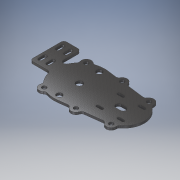
# Autodesk Inventor part: CAR REDUCTION PLATE I
Saved by Autodesk Inventor 2017 (Build 210142000, 142)
## iProperties
Part Number: CAR REDUCTION PLATE I
Material: Genérico
Document SubType Name: Modeling
Designer: Cristian
Density: 1 g/cm^3
Appearance: Valor por defecto
Author: Cristian
Autodesk Inventor part; units mm, degrees
ref_plane "YZ Plane" through (0, 0, 0) normal (1, 0, 0) x (0, 1, 0)
ref_plane "XZ Plane" through (0, 0, 0) normal (0, 1, 0) x (-1, 0, 0)
ref_plane "XY Plane" through (0, 0, 0) normal (0, 0, 1) x (1, 0, 0)
sketch "Boceto1" plane through (0, 0, 0) normal (0, 0, 1) x (1, 0, 0)
  circle A0 centre (0, 0) radius 57.15
  circle A1 centre (101.6, 0) radius 44.45
  circle A2 centre (-31.75, 47.519) radius 11.1125
  circle A3 centre (-31.75, -47.519) radius 11.1125
  circle A4 centre (114.3, 42.5971) radius 11.1125
  circle A5 centre (114.3, -42.5971) radius 11.1125
  line L0 (7.1437, 56.7018) -> (107.1562, 44.1014)
  circle A6 centre (44.45, 52.0016) radius 11.1125
  line L1 (7.1437, -56.7018) -> (107.1562, -44.1014)
  circle A7 centre (44.45, -52.0016) radius 11.1125
  dimension "d0" = 114.3
  dimension "d1" = 88.9
  dimension "d2" = 203.2
  dimension "d3" = 22.225
  dimension "d4" = 22.225
  dimension "d7" = 22.225
  dimension "d8" = 22.225
  dimension "d11" = 22.225
  dimension "d13" = 0
  dimension "d14" = 22.225
  dimension "d27" = 12.7
  dimension "d28" = 12.7
  dimension "d29" = 44.45
  dimension "d30" = 44.45
  dimension "d31" = 31.75
  dimension "d32" = 31.75
  constraints: 8 centre point, 8 point on circle, 4 end point, 4 tangent, 2 point on line, 1 coincident
  measures "d0" diameter of A0
  measures "d1" diameter of A1
  measures "d3" diameter of A2
  measures "d4" diameter of A3
  measures "d7" diameter of A4
  measures "d8" diameter of A5
  measures "d11" diameter of A6
  measures "d13" vertical distance of point (0, 0) A1.centre
  measures "d14" diameter of A7
  measures "d27" horizontal distance of A1.centre A4.centre
  measures "d28" horizontal distance of A1.centre A5.centre
  measures "d29" horizontal distance of point (0, 0) A6.centre
  measures "d30" horizontal distance of A7.centre point (0, 0)
  measures "d31" horizontal distance of point (0, 0) A2.centre
  measures "d32" horizontal distance of point (0, 0) A3.centre
extrude "Extrusión1" add sketch "Boceto1" along normal blind 5
sketch "Boceto2" plane through (0, 0, 5) normal (0, 0, 1) x (1, 0, 0)
  arc A0 (-21.9537, 52.7651) -> (-40.3458, 40.4764) centre (-31.75, 47.519) ccw projected
  circle A1 centre (-31.75, 47.519) radius 4.7625
  arc A2 (-40.3458, -40.4764) -> (-21.9537, -52.7651) centre (-31.75, -47.519) ccw projected
  circle A3 centre (-31.75, -47.519) radius 4.7625
  arc A4 (33.4247, -53.3907) -> (55.4753, -50.6125) centre (44.45, -52.0016) ccw projected
  circle A5 centre (44.45, -52.0016) radius 4.7625
  arc A6 (55.4753, 50.6125) -> (33.4247, 53.3907) centre (44.45, 52.0016) ccw projected
  circle A7 centre (44.45, 52.0016) radius 4.7625
  arc A8 (124.4689, 38.1158) -> (103.3657, 44.5789) centre (114.3, 42.5971) ccw projected
  circle A9 centre (114.3, 42.5971) radius 4.7625
  arc A10 (103.3657, -44.5789) -> (124.4689, -38.1158) centre (114.3, -42.5971) ccw projected
  circle A11 centre (114.3, -42.5971) radius 4.7625
  point P0 (0, 0)
  dimension "d18" = 9.525
  dimension "d19" = 9.525
  dimension "d20" = 9.525
  dimension "d21" = 9.525
  dimension "d22" = 9.525
  dimension "d23" = 9.525
  constraints: 6 centre point, 6 coincident
  measures "d18" diameter of A1
  measures "d19" diameter of A3
  measures "d20" diameter of A5
  measures "d21" diameter of A7
  measures "d22" diameter of A9
  measures "d23" diameter of A11
extrude "Extrusión2" cut sketch "Boceto2" against normal up to surface (5 mm away)
fillet "Empalme1" radius 6.35 12 edges at (-21.9537, -52.7651, 2.5) (-40.3458, -40.4764, 2.5) (33.4247, -53.3907, 2.5) (55.4753, -50.6125, 2.5) (124.4689, -38.1158, 2.5) (-40.3458, 40.4764, 2.5) (-21.9537, 52.7651, 2.5) (33.4247, 53.3907, 2.5) (55.4753, 50.6125, 2.5) (103.3657, 44.5789, 2.5) (124.4689, 38.1158, 2.5) (103.3657, -44.5789, 2.5)
sketch "Boceto3" plane through (0, 0, 0) normal (0, 0, -1) x (-1, 0, 0)
  circle A0 centre (0, 0) radius 7.1437
  circle A1 centre (0, -45) radius 6.35
  circle A2 centre (0, 45) radius 6.35
  line L0 (0, -45) -> (0, 0)
  line L1 (0, 0) -> (0, 45)
  dimension "d33" = 14.2875
  dimension "d34" = 12.7
  dimension "d35" = 12.7
  dimension "d36" = 45
  dimension "d37" = 45
  constraints: 4 end point, 3 centre point, 1 coincident, 1 collinear, 1 vertical
  measures "d33" diameter of A0
  measures "d34" diameter of A1
  measures "d35" diameter of A2
  measures "d36" distance of point (0, 0) L0.start
  measures "d37" distance of L1.end point (0, 0)
extrude "Extrusión3" cut sketch "Boceto3" against normal up to surface (5 mm away)
sketch "Boceto4" plane through (0, 0, 5) normal (0, 0, 1) x (1, 0, 0)
  circle A0 centre (93.4212, 0) radius 6.35
  line L0 (65.4212, -28) -> (121.4212, -28)
  line L1 (121.4212, -28) -> (121.4212, 28)
  line L2 (121.4212, 28) -> (65.4212, 28)
  line L3 (65.4212, 28) -> (65.4212, -28)
  line L4 (69.6712, -23.75) -> (117.1712, -23.75)
  line L5 (117.1712, -23.75) -> (117.1712, 23.75)
  line L6 (117.1712, 23.75) -> (69.6712, 23.75)
  line L7 (69.6712, 23.75) -> (69.6712, -23.75)
  circle A1 centre (74.8306, -23.75) radius 2.7781
  circle A2 centre (112.0118, -23.75) radius 2.7781
  circle A3 centre (122.3306, -23.75) radius 2.7781
  circle A4 centre (64.5118, -23.75) radius 2.7781
  line L8 (64.5118, -26.5281) -> (74.8306, -26.5281)
  line L9 (64.5118, -20.9719) -> (74.8306, -20.9719)
  line L10 (112.0118, -26.5281) -> (122.3306, -26.5281)
  line L11 (122.3306, -20.9719) -> (112.0118, -20.9719)
  circle A5 centre (74.8306, 23.75) radius 2.7781
  circle A6 centre (64.5118, 23.75) radius 2.7781
  line L12 (64.5118, 20.9719) -> (74.8306, 20.9719)
  line L13 (64.5118, 26.5281) -> (74.8306, 26.5281)
  circle A7 centre (112.0118, 23.75) radius 2.7781
  circle A8 centre (122.3306, 23.75) radius 2.7781
  line L14 (112.0118, 20.9719) -> (122.3306, 20.9719)
  line L15 (112.0118, 26.5281) -> (122.3306, 26.5281)
  circle A9 centre (98.5806, 0) radius 6.35
  circle A10 centre (88.2618, 0) radius 6.35
  line L16 (98.5806, 6.35) -> (88.2618, 6.35)
  line L17 (98.5806, -6.35) -> (88.2618, -6.35)
  point P0 (0, 0)
  dimension "d40" = 12.7
  dimension "d41" = 56
  dimension "d42" = 56
  dimension "d43" = 28
  dimension "d44" = 28
  dimension "d45" = 0
  dimension "d46" = 93.4212
  dimension "d47" = 47.5
  dimension "d48" = 47.5
  dimension "d49" = 23.75
  dimension "d50" = 23.75
  dimension "d57" = 5.5563
  dimension "d58" = 5.1594
  dimension "d59" = 5.5563
  dimension "d60" = 5.5563
  dimension "d61" = 5.1594
  dimension "d62" = 5.1594
  dimension "d63" = 5.5563
  dimension "d64" = 5.1594
  dimension "d65" = 0
  dimension "d66" = 5.5563
  dimension "d67" = 5.5563
  dimension "d68" = 5.1594
  dimension "d69" = 5.1594
  dimension "d70" = 0
  dimension "d71" = 5.5563
  dimension "d72" = 5.5563
  dimension "d73" = 5.1594
  dimension "d74" = 5.1594
  dimension "d75" = 0
  dimension "d78" = 12.7
  dimension "d79" = 12.7
  dimension "d80" = 5.1594
  dimension "d81" = 5.1594
  constraints: 36 end point, 20 point on circle, 20 tangent, 11 centre point, 5 point on line, 4 parallel, 2 horizontal, 2 perpendicular
  measures "d40" diameter of A0
  measures "d41" distance of L2.end L0.start
  measures "d42" distance of L1.end L2.end
  measures "d43" distance from line of L2 A0.centre
  measures "d44" distance from line of L3 A0.centre
  measures "d45" vertical distance of point (0, 0) A0.centre
  measures "d46" distance of point (0, 0) A0.centre
  measures "d47" distance of L6.end L4.start
  measures "d48" distance of L4.start L4.end
  measures "d49" distance from line of L4 A0.centre
  measures "d50" distance from line of L7 A0.centre
  measures "d57" diameter of A1
  measures "d58" distance of A1.centre L4.start
  measures "d59" diameter of A2
  measures "d60" diameter of A3
  measures "d61" distance of L4.end A2.centre
  measures "d62" distance of L4.end A3.centre
  measures "d63" diameter of A4
  measures "d64" distance of L4.start A4.centre
  measures "d65" distance from line of L4 A4.centre
  measures "d66" diameter of A5
  measures "d67" diameter of A6
  measures "d68" distance of L6.end A6.centre
  measures "d69" distance of L6.end A5.centre
  measures "d70" distance from line of L6 A6.centre
  measures "d71" diameter of A7
  measures "d72" diameter of A8
  measures "d73" distance of L5.end A7.centre
  measures "d74" distance of L5.end A8.centre
  measures "d75" distance from line of L6 A8.centre
  measures "d78" diameter of A9
  measures "d79" diameter of A10
  measures "d80" distance of A0.centre A9.centre
  measures "d81" distance of A0.centre A10.centre
extrude "Extrusión4" cut sketch "Boceto4" against normal up to next contours A0 A9 A10 | A0 A9 | A9 A10 A0 | A0 L16 A9 | A9 L17 A0 | A0 A10 A9 | A0 A10 L16 | A10 A9 | A9 A10 A0 | L17 A10 A0 | A0 A10 | L8 A4 L3 | L3 A4 L9 L7 L4 A1 L8 | L10 A2 L4 L5 L11 L1 A3 | L1 A3 L10 | A4 L3 | L3 A4 | A1 L4 | A3 L1 | L1 A3 | A2 L4 | A4 L9 L3 | L4 A1 | L4 L7 L9 A1 | L1 L11 A3 | A2 L11 L5 L4 | L4 A2 | L12 A6 L3 | L3 A6 L13 A5 L6 L7 L12 | L14 L5 L6 A7 L15 L1 A8 | L1 A8 L14 | A6 L3 | L3 A6 | L7 L6 A5 L12 | A8 L1 | L1 A8 | L14 A7 L6 L5 | A6 L13 L3 | A5 L6 | L1 L15 A8 | A7 L6 | A5 L6 | L6 A7
sketch "Boceto5" plane through (0, 0, 5) normal (0, 0, 1) x (1, 0, 0)
  line L0 (-101.6, -9.525) -> (-63.5, -9.525)
  line L1 (-63.5, -9.525) -> (-63.5, 66.675)
  line L2 (-63.5, 66.675) -> (-101.6, 66.675)
  line L3 (-101.6, 66.675) -> (-101.6, -9.525)
  arc A0 (127.9228, -35.8178) -> (127.9228, 35.8178) centre (101.6, 0) ccw projected
  line L4 (146.05, 0) -> (146.05, -41.4145)
  arc A1 (-17.8783, -54.2816) -> (7.1437, -56.7018) centre (0, 0) ccw projected
  line L5 (0, -57.15) -> (25.0965, -57.15)
  line L6 (-63.5, -9.525) -> (-38.1, -9.525)
  line L7 (-38.1, -9.525) -> (-38.1, 15.875)
  line L8 (-38.1, 15.875) -> (-63.5, 15.875)
  line L9 (-63.5, 15.875) -> (-63.5, -9.525)
  dimension "d82" = 247.65
  dimension "d83" = 76.2
  dimension "d84" = 123.825
  dimension "d85" = 38.1
  dimension "d86" = 25.4
  dimension "d87" = 25.4
  constraints: 20 end point, 4 parallel, 3 horizontal, 2 perpendicular, 2 point on circle, 1 tangent, 1 vertical
  measures "d82" distance between parallel lines of L4 L3
  measures "d83" distance of L2.end L0.start
  measures "d84" distance from line of L5.start L2
  measures "d85" distance of L1.end L2.end
  measures "d86" distance of L8.end L7.end
  measures "d87" distance of L7.end L6.end
extrude "Extrusión5" add sketch "Boceto5" against normal up to surface (5 mm away)
fillet "Empalme2" radius 6.35 6 edges at (-101.6, 66.675, 2.5) (-63.5, 66.675, 2.5) (-101.6, -9.525, 2.5) (-56.3507, -9.525, 2.5) (-54.9009, 15.875, 2.5) (-63.5, 15.875, 2.5)
sketch "Boceto6" plane through (0, 0, 5) normal (0, 0, 1) x (1, 0, 0)
  circle A0 centre (-73.5648, 48.4188) radius 3.9687
  line L0 (-69.85, 66.675) -> (-95.25, 66.675) projected
  line L1 (-63.5, 27.679) -> (-63.5, 60.325) projected
  circle A1 centre (-73.5648, 53.975) radius 3.9688
  circle A2 centre (-73.5648, 42.8625) radius 3.9687
  line L2 (-69.596, 53.975) -> (-69.596, 42.8625)
  line L3 (-77.5335, 53.975) -> (-77.5335, 42.8625)
  circle A3 centre (-91.5353, 48.4188) radius 3.9687
  line L4 (-101.6, 60.325) -> (-101.6, -3.175) projected
  circle A4 centre (-91.5353, 53.975) radius 3.9687
  circle A5 centre (-91.5353, 42.8625) radius 3.9687
  line L5 (-87.5665, 53.975) -> (-87.5665, 42.8625)
  line L6 (-95.504, 53.975) -> (-95.504, 42.8625)
  circle A6 centre (-73.5648, 8.7312) radius 3.9688
  line L7 (-95.25, -9.525) -> (-61.4836, -9.525) projected
  circle A7 centre (-73.5648, 3.175) radius 3.9688
  circle A8 centre (-73.5648, 14.2875) radius 3.9687
  line L8 (-69.596, 14.2875) -> (-69.596, 3.175)
  line L9 (-77.5335, 3.175) -> (-77.5335, 14.2875)
  circle A9 centre (-91.5353, 8.7312) radius 3.9688
  circle A10 centre (-91.5353, 3.175) radius 3.9688
  circle A11 centre (-91.5353, 14.2875) radius 3.9688
  line L10 (-87.5665, 14.2875) -> (-87.5665, 3.175)
  line L11 (-95.504, 3.175) -> (-95.504, 14.2875)
  point P0 (0, 0)
  dimension "d91" = 7.9375
  dimension "d92" = 18.2563
  dimension "d93" = 10.0648
  dimension "d94" = 7.9375
  dimension "d95" = 7.9375
  dimension "d96" = 5.5563
  dimension "d97" = 5.5563
  dimension "d98" = 0
  dimension "d99" = 0
  dimension "d100" = 7.9375
  dimension "d101" = 10.0648
  dimension "d102" = 18.2563
  dimension "d103" = 7.9375
  dimension "d104" = 7.9375
  dimension "d105" = 5.5563
  dimension "d106" = 5.5563
  dimension "d107" = 0
  dimension "d108" = 0
  dimension "d109" = 7.9375
  dimension "d110" = 18.2563
  dimension "d111" = 10.0648
  dimension "d112" = 7.9375
  dimension "d113" = 7.9375
  dimension "d114" = 5.5563
  dimension "d115" = 5.5563
  dimension "d116" = 0
  dimension "d117" = 0
  dimension "d118" = 7.9375
  dimension "d119" = 18.2563
  dimension "d120" = 10.0648
  dimension "d121" = 7.9375
  dimension "d122" = 7.9375
  dimension "d123" = 5.5563
  dimension "d124" = 5.5563
  dimension "d125" = 0
  dimension "d126" = 0
  constraints: 16 end point, 16 point on circle, 15 tangent, 12 centre point, 1 parallel
  measures "d91" diameter of A0
  measures "d92" distance from line of L0 A0.centre
  measures "d93" distance from line of L1 A0.centre
  measures "d94" diameter of A1
  measures "d95" diameter of A2
  measures "d96" distance of A0.centre A1.centre
  measures "d97" distance of A2.centre A0.centre
  measures "d98" horizontal distance of A0.centre A1.centre
  measures "d99" horizontal distance of A0.centre A2.centre
  measures "d100" diameter of A3
  measures "d101" distance from line of A3.centre L4
  measures "d102" distance from line of L0 A3.centre
  measures "d103" diameter of A4
  measures "d104" diameter of A5
  measures "d105" distance of A3.centre A4.centre
  measures "d106" distance of A5.centre A3.centre
  measures "d107" horizontal distance of A3.centre A4.centre
  measures "d108" horizontal distance of A3.centre A5.centre
  measures "d109" diameter of A6
  measures "d110" distance from line of L7 A6.centre
  measures "d111" distance from line of L1 A6.centre
  measures "d112" diameter of A7
  measures "d113" diameter of A8
  measures "d114" distance of A6.centre A8.centre
  measures "d115" distance of A6.centre A7.centre
  measures "d116" horizontal distance of A6.centre A8.centre
  measures "d117" horizontal distance of A6.centre A7.centre
  measures "d118" diameter of A9
  measures "d119" distance from line of L7 A9.centre
  measures "d120" distance from line of L4 A9.centre
  measures "d121" diameter of A10
  measures "d122" diameter of A11
  measures "d123" distance of A9.centre A11.centre
  measures "d124" distance of A10.centre A9.centre
  measures "d125" horizontal distance of A9.centre A11.centre
  measures "d126" horizontal distance of A9.centre A10.centre
extrude "Extrusión6" cut sketch "Boceto6" against normal up to next
equation "\"d16\" = t"
equation "\"d18\" = Q"
equation "\"d19\" = Q"
equation "\"d20\" = Q"
equation "\"d21\" = Q"
equation "\"d22\" = Q"
equation "\"d23\" = Q"
equation "\"d33\" = DF"
equation "\"d34\" = NF"
equation "\"d35\" = NF"
equation "\"d36\" = 0.5 * JF"
equation "\"d37\" = 0.5 * JF"
equation "\"d40\" = DM"
equation "\"d41\" = AM"
equation "\"d42\" = AM"
equation "\"d43\" = 0.5 * AM"
equation "\"d44\" = 0.5 * AM"
equation "\"d46\" = CM"
equation "\"d47\" = BM"
equation "\"d48\" = BM"
equation "\"d49\" = 0.5 * BM"
equation "\"d50\" = 0.5 * BM"
equation "\"d57\" = NM"
equation "\"d59\" = NM"
equation "\"d60\" = NM"
equation "\"d63\" = NM"
equation "\"d66\" = NM"
equation "\"d67\" = NM"
equation "\"d71\" = NM"
equation "\"d72\" = NM"
equation "\"d78\" = DM"
equation "\"d79\" = DM"
equation "\"d91\" = DH"
equation "\"d94\" = DH"
equation "\"d95\" = DH"
equation "\"d100\" = DH"
equation "\"d103\" = DH"
equation "\"d104\" = DH"
equation "\"d109\" = DH"
equation "\"d112\" = DH"
equation "\"d113\" = DH"
equation "\"d118\" = DH"
equation "\"d121\" = DH"
equation "\"d122\" = DH"
equation "\"t\" = 5"
equation "\"Q\" = 9.525"
equation "\"DF\" = 14.2875"
equation "\"NF\" = 12.7"
equation "\"DM\" = 12.7"
equation "\"NM\" = 5.55625"
equation "\"CM\" = 93.4212"
equation "\"AM\" = 56"
equation "\"BM\" = 47.5"
equation "\"DH\" = 7.9375"
equation "\"JF\" = 90"
